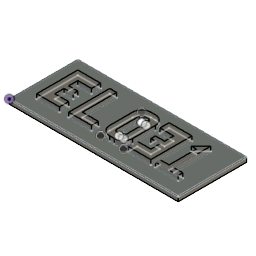
MILL EL 031 (Autodesk Fusion 360 design; units mm, degrees)
part number: 2026-06-20-13-13-11-387
Autodesk Fusion 360 part; units mm, degrees
sketch "Sketch1" plane through (0, 0, 0) normal (0, 0, 1) x (1, 0, 0)
  line L0 (0, 0) -> (37, 0)
  line L1 (37, 0) -> (37, 15)
  line L2 (37, 15) -> (0, 15)
  line L3 (0, 15) -> (0, 0)
  line L4 (3, 12) -> (3, 3)
  line L5 (3, 3) -> (8, 3)
  line L6 (8, 3) -> (8, 5)
  line L7 (8, 5) -> (5, 5)
  line L8 (5, 5) -> (5, 7)
  line L9 (5, 7) -> (7, 7)
  line L10 (7, 7) -> (7, 8)
  line L11 (7, 8) -> (5, 8)
  line L12 (5, 8) -> (5, 10)
  line L13 (5, 10) -> (8, 10)
  line L14 (8, 10) -> (8, 12)
  line L15 (8, 12) -> (3, 12)
  line L16 (10, 12) -> (10, 3)
  line L17 (10, 3) -> (15, 3)
  line L18 (15, 3) -> (15, 4.5)
  line L19 (15, 4.5) -> (11.5, 4.5)
  line L20 (11.5, 4.5) -> (11.5, 12)
  line L21 (11.5, 12) -> (10, 12)
  line L22 (19, 12) -> (20, 12)
  line L23 (22, 10) -> (22, 5)
  line L24 (20, 3) -> (19, 3)
  line L25 (17, 5) -> (17, 10)
  line L26 (19, 10.5) -> (20, 10.5)
  line L27 (20.5, 10) -> (20.5, 5)
  line L28 (20, 4.5) -> (19, 4.5)
  line L29 (18.5, 5) -> (18.5, 10)
  line L30 (23, 12) -> (28, 12)
  line L31 (28, 12) -> (28, 3)
  line L32 (28, 3) -> (23, 3)
  line L33 (23, 5) -> (23, 3)
  line L34 (23, 5) -> (26, 5)
  line L35 (26, 5) -> (26, 7)
  line L36 (26, 7) -> (24, 7)
  line L37 (24, 7) -> (24, 8)
  line L38 (24, 8) -> (26, 8)
  line L39 (26, 8) -> (26, 10)
  line L40 (26, 10) -> (23, 10)
  line L41 (23, 10) -> (23, 12)
  line L42 (32, 12.1213) -> (29.8787, 10)
  line L43 (29.8787, 10) -> (31, 10)
  line L44 (31, 10) -> (31, 4)
  line L45 (31, 4) -> (29, 4)
  line L46 (29, 4) -> (29, 3)
  line L47 (29, 3) -> (34, 3)
  line L48 (34, 3) -> (34, 4)
  line L49 (34, 4) -> (32, 4)
  line L50 (32, 4) -> (32, 12.1213)
  arc A0 (19, 12) -> (17, 10) centre (19, 10) ccw
  arc A1 (22, 10) -> (20, 12) centre (20, 10) ccw
  arc A2 (20, 3) -> (22, 5) centre (20, 5) ccw
  arc A3 (17, 5) -> (19, 3) centre (19, 5) ccw
  arc A4 (19, 10.5) -> (18.5, 10) centre (19, 10) ccw
  arc A5 (20.5, 10) -> (20, 10.5) centre (20, 10) ccw
  arc A6 (20, 4.5) -> (20.5, 5) centre (20, 5) ccw
  arc A7 (18.5, 5) -> (19, 4.5) centre (19, 5) ccw
  point P0 (17, 12)
  point P1 (22, 3)
  point P2 (17, 3)
  dimension "d1" = 37
  dimension "d2" = 15
  dimension "d3" = 9
  dimension "d4" = 5
  dimension "d5" = 3
  dimension "d6" = 3
  dimension "d7" = 2
  dimension "d8" = 2
  dimension "d9" = 2
  dimension "d10" = 2
  dimension "d11" = 5
  dimension "d12" = 4
  dimension "d13" = 2
  dimension "d14" = 2
  dimension "d15" = 2
  dimension "d16" = 9
  dimension "d17" = 3
  dimension "d18" = 5
  dimension "d19" = 3.5
  dimension "d20" = 7.5
  dimension "d21" = 2
  dimension "d22" = 3
  dimension "d23" = 5
  dimension "d24" = 9
  dimension "d25" = 2
  dimension "d26" = 2
  dimension "d27" = 2
  dimension "d28" = 2
  dimension "d29" = 1.5
  dimension "d30" = 1.5
  dimension "d31" = 1.5
  dimension "d32" = 1.5
  dimension "d33" = 0.5
  dimension "d34" = 1
  dimension "d35" = 3
  dimension "d36" = 9
  dimension "d37" = 2
  dimension "d38" = 2
  dimension "d39" = 5
  dimension "d40" = 1
  dimension "d41" = 2
  dimension "d42" = 2
  dimension "d43" = 2
  dimension "d44" = 2
  dimension "d45" = 4
  dimension "d46" = 5
  dimension "d47" = 3
  dimension "d48" = 1
  dimension "d49" = 2
  dimension "d50" = 2
  dimension "d51" = 1
  dimension "d52" = 1
  dimension "d53" = 45
  dimension "d54" = 6
  dimension "d55" = 3
  dimension "d56" = 0.5
  constraint horizontal L0
  constraint vertical L1
  constraint horizontal L2
  constraint vertical L3
  constraint coincident L0.start L3.end
  constraint perpendicular L2 L4
  constraint perpendicular L4 L5
  constraint perpendicular L5 L6
  constraint perpendicular L6 L7
  constraint perpendicular L7 L8
  constraint perpendicular L8 L9
  constraint perpendicular L9 L10
  constraint perpendicular L10 L11
  constraint perpendicular L11 L12
  constraint perpendicular L12 L13
  constraint perpendicular L13 L14
  constraint perpendicular L4 L15
  constraint perpendicular L13 L16
  constraint perpendicular L14 L17
  constraint perpendicular L13 L18
  constraint perpendicular L14 L19
  constraint perpendicular L19 L20
  constraint perpendicular L16 L21
  constraint horizontal L22
  constraint vertical L23
  constraint horizontal L24
  constraint vertical L25
  constraint horizontal L26
  constraint vertical L27
  constraint horizontal L28
  constraint vertical L29
  constraint parallel L2 L30
  constraint perpendicular L30 L31
  constraint perpendicular L31 L32
  constraint perpendicular L32 L33
  constraint perpendicular L33 L34
  constraint perpendicular L34 L35
  constraint perpendicular L35 L36
  constraint perpendicular L36 L37
  constraint perpendicular L37 L38
  constraint perpendicular L38 L39
  constraint perpendicular L23 L40
  constraint perpendicular L30 L41
  constraint perpendicular L31 L43
  constraint perpendicular L43 L44
  constraint perpendicular L44 L45
  constraint perpendicular L45 L46
  constraint perpendicular L46 L47
  constraint perpendicular L47 L48
  constraint perpendicular L48 L49
  constraint perpendicular L49 L50
  constraint coincident P0 L22
  constraint coincident P0 L25
  constraint tangent L22 A0
  constraint tangent L25 A0
  constraint tangent L22 A1
  constraint tangent L23 A1
  constraint coincident P1 L23
  constraint coincident P1 L24
  constraint tangent L23 A2
  constraint tangent L24 A2
  constraint coincident P2 L24
  constraint coincident P2 L25
  constraint tangent L24 A3
  constraint tangent L25 A3
  constraint tangent L26 A4
  constraint tangent L29 A4
  constraint tangent L26 A5
  constraint tangent L27 A5
  constraint equal A4 A5
  constraint tangent L27 A6
  constraint tangent L28 A6
  constraint equal A4 A6
  constraint tangent L28 A7
  constraint tangent L29 A7
  measures "d1" distance of L0.start L0.end
  measures "d2" distance of L0.start L2.end
  measures "d3" distance of L4.start L4.end
  measures "d4" distance of L4.end L5.end
  measures "d5" distance of L3 L4
  measures "d6" distance of L0 L5
  measures "d7" distance of L5 L7
  measures "d8" distance of L13 L15
  measures "d9" distance of L11 L13
  measures "d10" distance of L8.end L9.end
  measures "d11" distance of L4 L14
  measures "d12" distance of L4 L10
  measures "d13" distance of L4 L12
  measures "d14" distance of L7 L9
  measures "d15" distance of L6 L16
  measures "d16" distance of L16.start L16.end
  measures "d17" distance of L0 L17
  measures "d18" distance of L16.end L17.end
  measures "d19" distance of L18.end L19.end
  measures "d20" distance of L19.end L20.end
  measures "d21" distance of L18 L25
  measures "d22" distance of L0 L24
  measures "d23" distance of P1 P2
  measures "d24" distance of P0 P2
  measures "d25" radius of A0
  measures "d26" radius of A1
  measures "d27" radius of A2
  measures "d28" radius of A3
  measures "d29" distance of L25 L29
  measures "d30" distance of L22 L26
  measures "d31" distance of L23 L27
  measures "d32" distance of L24 L28
  measures "d33" radius of A4
  measures "d34" distance of L23 L33
  measures "d35" distance of L0 L32
  measures "d36" distance of L30.end L31.end
  measures "d37" distance of L32 L34
  measures "d38" distance of L30 L40
  measures "d39" distance of L31 L41
  measures "d40" distance of L23 L41
  measures "d41" distance of L31 L39
  measures "d42" distance of L31 L35
  measures "d43" distance of L34 L36
  measures "d44" distance of L38 L40
  measures "d45" distance of L31 L37
  measures "d46" distance of L46.end L47.end
  measures "d47" distance of L0 L47
  measures "d48" distance of L31 L46
  measures "d49" distance of L44.end L45.end
  measures "d50" distance of L48.end L49.end
  measures "d51" distance of L47 L49
  measures "d52" distance of L45 L47
  measures "d53" angle of L42 L50
  measures "d54" distance of L43 L45
  measures "d55" distance of L42.start L42.end
  measures "d56" radius of A7
extrude "Extrude1" add sketch "Sketch1" against normal blind 1 makes body 1 at (34.3333, 10.3738, 0) makes body 2 at (19.8333, 8.3333, 0)
extrude "Extrude2" add sketch "Sketch1" along normal blind 1 separate body contours L4 L5 L6 L7 L8 L9 L10 L11 L12 L13 L14 L15 | L16 L17 L18 L19 L20 L21 | L22 L23 L24 L25 A0 A1 A2 A3 | L30 L31 L32 L33 L34 L35 L36 L37 L38 L39 L40 L41 | L42 L43 L44 L45 L46 L47 L48 L49 L50 makes body 3 at (17.5, 6.6667, 0) makes body 4 at (10.5, 6.5, 0) makes body 5 at (27.3333, 7.6667, 0) makes body 6 at (3.6667, 7.6667, 0) makes body 7 at (31.6667, 8.7071, 0)
